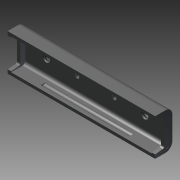
# Autodesk Inventor part: BSPG1560 Table
Saved by Autodesk Inventor 2016 (Build 200138000, 138)
## iProperties
Category: PARTsolutions
Company: IKO
Created: 2015-05-07
Part Number: BSPG1560 Table
Catalog Web Link: www.cadenas.de
Description: BSPG- Table-
Vendor: IKO
Document SubType Name: Modeling
Designer: PARTuser1
Manufacturer: IKO
Mass: 1.76636 g
Surface Area: 33.173 cm^2
Volume: 1.76636 cm^3
Density: 1 g/cm^3
Material: Generic
Appearance: PSOLRGB-192-192-192
PSOL_IDENT_0: {$CADENAS_DATA\23d-libs\iko\linear_way_series\precise_ball_slide\bspg_1.prj},175 {VTYP=3D},{NB=BSPG1
PSOL_IDENT_1: 560 Table},{LINA=BSPG1560 Table},{NN=BSPG- Table},{DATE=16.12.2009 04:05:19},{GEOMDATE=16.12.2009 04
PSOL_IDENT_2: :05:00},{VERSION=},{LINEID=60},{LINESUBID=-1},{WBVAR=}  {NB=BSPG1560 Table},{LINA=BSPG1560 Table},{K
PSOL_IDENT_3: T=DUMMY},{IDNR=},{TP=BSPG},{SZ=15},{W=15.000},{H=8.000},{L=60.000},{MS=40.000},{L1=40.000},{M1=3.000
PSOL_IDENT_4: },{S1=2.500},{SH1=7.000},{ST1=1.200},{LB=57.000},{SW=9.600},{L2=40.000},{M2=3.000},{S2=3.000},{SH2=4
PSOL_IDENT_5: .500},{ST2=1.200},{R=2.790},{R1=1.300},{W2=5.800},{ST3=2.000},{T1=1.400},{LN=15.100},{DN=1.800},{LX=
PSOL_IDENT_6: 36.000},{RZ=0.300},{DA=2.200}
SUPPLIER: IKO
ARTICLENO: BSPG1560 Table
BOMINFO: BSPG1560 Table
CREATOR: CADENAS GmbH
Title: BSPG1560 Table
Author: Cadenas PARTsolutions
Autodesk Inventor part; units mm, degrees
ref_plane "YZ Plane" through (0, 0, 0) normal (1, 0, 0) x (0, 1, 0)
ref_plane "XZ Plane" through (0, 0, 0) normal (0, 1, 0) x (-1, 0, 0)
ref_plane "XY Plane" through (0, 0, 0) normal (0, 0, 1) x (1, 0, 0)
sketch "Sketch_1" plane through (0, 0, 0) normal (1, 0, 0) x (0, 1, 0)
  line L0 (-7, 7.5) -> (-7, 6.3)
  line L1 (-7, 6.3) -> (-2.5, 6.3)
  arc A0 (-1.2, 5) -> (-2.5, 6.3) centre (-2.5, 5) ccw
  line L2 (-1.2, 5) -> (-1.2, -5)
  arc A1 (-2.5, -6.3) -> (-1.2, -5) centre (-2.5, -5) ccw
  line L3 (-2.5, -6.3) -> (-7, -6.3)
  line L4 (-7, -6.3) -> (-7, -7.5)
  line L5 (-7, -7.5) -> (-2.79, -7.5)
  arc A2 (-2.79, -7.5) -> (0, -4.71) centre (-2.79, -4.71) ccw
  line L6 (0, -4.71) -> (0, 4.71)
  arc A3 (0, 4.71) -> (-2.79, 7.5) centre (-2.79, 4.71) ccw
  line L7 (-2.79, 7.5) -> (-7, 7.5)
  constraints: 16 end point, 8 point on circle, 4 centre point
extrude "Extrusion1" add sketch "Sketch_1" along normal blind 60
sketch "Sketch_2" plane through (0.02, 0, 0) normal (1, 0, 0) x (0, 0, -1)
  line L0 (-6.3, -7) -> (-5.95, -7)
  line L1 (-5.95, -7) -> (-5.6669, -3.9266)
  arc A0 (-4.8703, -3.2) -> (-5.6669, -3.9266) centre (-4.8703, -4) ccw
  line L2 (-4.8703, -3.2) -> (4.8703, -3.2)
  arc A1 (5.6669, -3.9266) -> (4.8703, -3.2) centre (4.8703, -4) ccw
  line L3 (5.6669, -3.9266) -> (5.95, -7)
  line L4 (5.95, -7) -> (6.3, -7)
  line L5 (6.3, -7) -> (6.3, -2.5)
  arc A2 (6.3, -2.5) -> (5, -1.2) centre (5, -2.5) ccw
  line L6 (5, -1.2) -> (-5, -1.2)
  arc A3 (-5, -1.2) -> (-6.3, -2.5) centre (-5, -2.5) ccw
  line L7 (-6.3, -2.5) -> (-6.3, -7)
  constraints: 16 end point, 8 point on circle, 4 centre point
extrude "Extrusion2" add sketch "Sketch_2" along normal blind 1.4
sketch "Sketch_3" plane through (59.98, 0, 0) normal (1, 0, 0) x (0, 0, -1)
  line L0 (-6.3, -7) -> (-5.95, -7)
  line L1 (-5.95, -7) -> (-5.6669, -3.9266)
  arc A0 (-4.8703, -3.2) -> (-5.6669, -3.9266) centre (-4.8703, -4) ccw
  line L2 (-4.8703, -3.2) -> (4.8703, -3.2)
  arc A1 (5.6669, -3.9266) -> (4.8703, -3.2) centre (4.8703, -4) ccw
  line L3 (5.6669, -3.9266) -> (5.95, -7)
  line L4 (5.95, -7) -> (6.3, -7)
  line L5 (6.3, -7) -> (6.3, -2.5)
  arc A2 (6.3, -2.5) -> (5, -1.2) centre (5, -2.5) ccw
  line L6 (5, -1.2) -> (-5, -1.2)
  arc A3 (-5, -1.2) -> (-6.3, -2.5) centre (-5, -2.5) ccw
  line L7 (-6.3, -2.5) -> (-6.3, -7)
  constraints: 16 end point, 8 point on circle, 4 centre point
extrude "Extrusion3" add sketch "Sketch_3" against normal blind 1.4
sketch "Sketch_4" plane through (10, 0, 0) normal (1, 0, 0) x (0, 0, -1)
  line L0 (0, -1.2) -> (0, 0)
  line L1 (0, 0) -> (1.5, 0)
  line L2 (1.5, 0) -> (1.2295, -0.2705)
  line L3 (1.2295, -0.2705) -> (1.2295, -0.9295)
  line L4 (1.2295, -0.9295) -> (1.5, -1.2)
  line L5 (1.5, -1.2) -> (0, -1.2)
  line L6 (0, -1.2) -> (0, 0)
  constraints: 14 end point
revolve "Revolution1" cut sketch "Sketch_4" angle 360 about axis through (10, -1.2, 0) along (0, -1, 0)
thread "Thread1" size "M3x0.5" class "6H" standard "ISO Metric profile" full length
sketch "Sketch_5" plane through (50, 0, 0) normal (1, 0, 0) x (0, 0, -1)
  line L0 (0, -1.2) -> (0, 0)
  line L1 (0, 0) -> (1.5, 0)
  line L2 (1.5, 0) -> (1.2295, -0.2705)
  line L3 (1.2295, -0.2705) -> (1.2295, -0.9295)
  line L4 (1.2295, -0.9295) -> (1.5, -1.2)
  line L5 (1.5, -1.2) -> (0, -1.2)
  line L6 (0, -1.2) -> (0, 0)
  constraints: 14 end point
revolve "Revolution2" cut sketch "Sketch_5" angle 360 about axis through (50, -1.2, 0) along (0, -1, 0)
thread "Thread2" size "M3x0.5" class "6H" standard "ISO Metric profile" full length
sketch "Sketch6" plane through (1.42, -1.2, -5) normal (0, -1, 0) x (1, 0, 0)
  point P0 (36.13, 5)
hole "Hole1" at (37.55, -1.2, 0) direction (0, 1, 0) diameter 1.8 depth 1.2
sketch "Sketch7" plane through (1.42, -1.2, -5) normal (0, -1, 0) x (1, 0, 0)
  point P0 (21.03, 5)
hole "Hole2" at (22.45, -1.2, 0) direction (0, 1, 0) diameter 1.8 depth 1.2
sketch "Sketch_9" plane through (30, 0, 0) normal (1, 0, 0) x (0, 0, -1)
  arc A0 (-5.75, -3.5) -> (-5.75, -5.7) centre (-5.75, -4.6) ccw
  line L0 (-5.75, -5.7) -> (-5.75, -3.5)
  constraints: 2 end point, 2 point on circle, 1 centre point
extrude "Extrusion4" cut sketch "Sketch_9" along normal mid plane 36
sketch "Sketch_10" plane through (30, 0, 0) normal (1, 0, 0) x (0, 0, -1)
  line L0 (5.75, -3.5) -> (5.75, -5.7)
  arc A0 (5.75, -5.7) -> (5.75, -3.5) centre (5.75, -4.6) ccw
  constraints: 2 end point, 2 point on circle, 1 centre point
extrude "Extrusion5" cut sketch "Sketch_10" along normal mid plane 36
ref_plane "bspg_1_XY" through (30, -4.6, 0) normal (1, 0, 0) x (0, 0, -1)
ref_plane "bspg_1_YZ" through (30, -4.6, 0) normal (0, 0, -1) x (0, 1, 0)
ref_plane "bspg_1_ZX" through (30, -4.6, 0) normal (0, 1, 0) x (1, 0, 0)
ref_plane "bspg_1r_XY" through (30, -3.5, 0) normal (1, 0, 0) x (0, 0, -1)
ref_plane "bspg_1r_YZ" through (30, -3.5, 0) normal (0, 0, -1) x (0, 1, 0)
ref_plane "bspg_1r_ZX" through (30, -3.5, 0) normal (0, 1, 0) x (1, 0, 0)
ref_plane "bspg_d_XY" through (0, 0, 0) normal (0, 1, 0) x (1, 0, 0)
ref_plane "bspg_d_YZ" through (0, 0, 0) normal (1, 0, 0) x (0, 0, -1)
ref_plane "bspg_d_ZX" through (0, 0, 0) normal (0, 0, -1) x (0, 1, 0)
body "Solid1"
